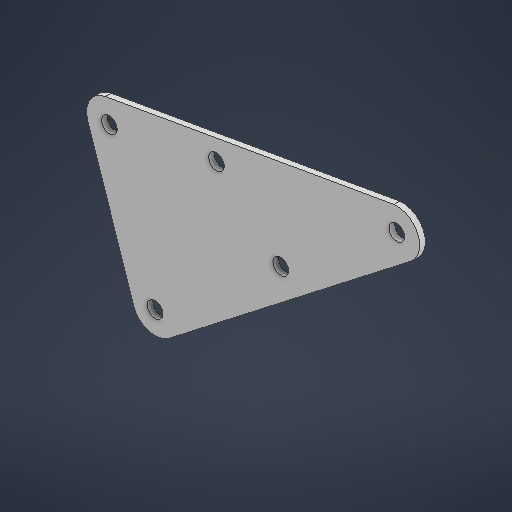
# Autodesk Inventor part: Lbsupportpoly
Saved by Autodesk Inventor 2025.2 (Build 292293000, 293)
## iProperties
Created: 2025-03-29
Part Number: Lbsupportpoly
Material: Generic
Document SubType Name: Modeling
Designer: roejo
Density: 1 g/cm^3
Appearance: Default
Author: roejo
Autodesk Inventor part; units mm, degrees
ref_plane "YZ Plane" through (0, 0, 0) normal (1, 0, 0) x (0, 1, 0)
ref_plane "XZ Plane" through (0, 0, 0) normal (0, 1, 0) x (-1, 0, 0)
ref_plane "XY Plane" through (0, 0, 0) normal (0, 0, 1) x (1, 0, 0)
sketch "Sketch2" plane through (0, 0, 0) normal (0, 0, 1) x (1, 0, 0)
  circle A0 centre (-9.8721, 18.0152) radius 2.1844
  circle A1 centre (40.2822, 26.089) radius 2.1844
  circle A2 centre (-26.9412, -26.089) radius 2.1844
  circle A3 centre (-39.6412, 12.011) radius 2.1844
  circle A4 centre (8.0053, 1.7888) radius 2.1844
  circle A5 centre (40.2822, 26.089) radius 6.35
  circle A6 centre (-26.9412, -26.089) radius 6.35
  line L0 (44.2198, 21.1073) -> (-23.0477, -31.1053)
  circle A7 centre (-39.6412, 12.011) radius 6.35
  line L1 (-32.9918, -28.0161) -> (-45.6653, 10.0028)
  line L2 (39.4559, 32.385) -> (-40.7423, 18.2648)
  point P0 (0, 0)
  dimension "d12" = 12.7
  dimension "d13" = 12.7
  dimension "d14" = 12.7
  constraints: 8 centre point, 6 end point, 6 point on circle, 3 coincident, 3 tangent
  measures "d12" diameter of A5
  measures "d13" diameter of A6
  measures "d14" diameter of A7
extrude "Extrusion2" add sketch "Sketch2" along normal blind 1.5875 contours A5 L0 A6 L1 A7 L2 | A6 | A7
body "Solid2"
